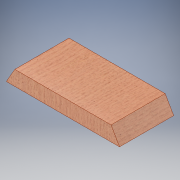
# Autodesk Inventor part: BA01
Saved by Autodesk Inventor 2017 (Build 210142000, 142)
## iProperties
Created: 2018-10-17
Part Number: BA01
Material: Wood (Oak)
Document SubType Name: Modeling
Designer: Administrator
Density: 0.76 g/cm^3
Appearance: White Oak - Natural Medium Gloss
Author: Administrator
Autodesk Inventor part; units mm, degrees
ref_plane "YZ Plane" through (0, 0, 0) normal (1, 0, 0) x (0, 1, 0)
ref_plane "XZ Plane" through (0, 0, 0) normal (0, 1, 0) x (-1, 0, 0)
ref_plane "XY Plane" through (0, 0, 0) normal (0, 0, 1) x (1, 0, 0)
sketch "Sketch1" plane through (0, 0, 0) normal (0, 0, 1) x (1, 0, 0)
  line L0 (0, 0) -> (292.1, 0)
  line L1 (0, 0) -> (21.997, 38.1)
  line L2 (21.997, 38.1) -> (270.103, 38.1)
  line L3 (270.103, 38.1) -> (292.1, 0)
  dimension "d1" = 292.1
  dimension "d2" = 38.1
  dimension "d3" = 60
  dimension "d4" = 60
  constraints: 8 end point, 2 horizontal, 1 coincident
  measures "d1" distance of L0.start L0.end
  measures "d2" distance between parallel lines of L0 L2
  measures "d3" angle of L0 L1
  measures "d4" angle of L0 L3
extrude "Extrusion1" add sketch "Sketch1" along normal blind 139.7
body "Solid1"
